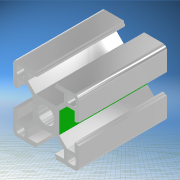
# Autodesk Inventor part: 30x30 aluminum
Saved by Autodesk Inventor 2020.2 (Build 242310000, 310)
## iProperties
Created: 2019-10-26
Part Number: 30x30 aluminum
Material: Aluminum 6061
Document SubType Name: Modeling
Designer: Sunoj
Density: 2.7 g/cm^3
Appearance: Aluminum - Flat
Mass: 340.698 g
Surface Area: 1270.55 cm^2
Volume: 126.184 cm^3
d0: 40.000 mm
Author: Sunoj
Autodesk Inventor part; units mm, degrees
ref_plane "YZ Plane" through (0, 0, 0) normal (1, 0, 0) x (0, 1, 0)
ref_plane "XZ Plane" through (0, 0, 0) normal (0, 1, 0) x (-1, 0, 0)
ref_plane "XY Plane" through (0, 0, 0) normal (0, 0, 1) x (1, 0, 0)
sketch "Sketch1" plane through (0, 0, 0) normal (0, 0, 1) x (1, 0, 0)
  line L0 (-4.1, 13) -> (-4.1, 14)
  line L1 (-4.1, 14) -> (-4.6, 14)
  line L2 (-4.6, 14) -> (-4.6, 15)
  line L3 (-4.6, 14) -> (-4.6, 15)
  line L4 (-4.6, 15) -> (-13, 15)
  arc A0 (-13, 15) -> (-15, 13) centre (-13, 13) ccw
  line L5 (-15, 13) -> (-15, 4.6)
  line L6 (-15, 13) -> (-15, 4.6)
  line L7 (-15, 4.6) -> (-14, 4.6)
  line L8 (-15, 4.6) -> (-14, 4.6)
  line L9 (-14, 4.6) -> (-14, 4.1)
  line L10 (-14, 4.6) -> (-14, 4.1)
  line L11 (-14, 4.1) -> (-13, 4.1)
  line L12 (-13, 4.1) -> (-13, 8.25)
  line L13 (-13, 8.25) -> (-9.5, 8.25)
  line L14 (-13, 8.25) -> (-9.5, 8.25)
  line L15 (-9.5, 8.25) -> (-6, 4.75)
  line L16 (-6, 4.75) -> (-6, -4.75)
  line L17 (-6, 4.75) -> (-6, -4.75)
  line L18 (-6, -4.75) -> (-9.5, -8.25)
  line L19 (-14, -4.1) -> (-13, -4.1)
  line L20 (-13, -4.1) -> (-14, -4.1)
  line L21 (-14, -4.6) -> (-14, -4.1)
  line L22 (-14, -4.1) -> (-14, -4.6)
  line L23 (-15, -4.6) -> (-14, -4.6)
  line L24 (-14, -4.6) -> (-15, -4.6)
  line L25 (-8.25, 13) -> (-4.1, 13)
  line L26 (-4.1, 13) -> (-8.25, 13)
  line L27 (-8.25, 9.5) -> (-8.25, 13)
  line L28 (-8.25, 13) -> (-8.25, 9.5)
  line L29 (-4.75, 6) -> (-8.25, 9.5)
  line L30 (-8.25, 9.5) -> (-4.75, 6)
  line L31 (4.75, 6) -> (-4.75, 6)
  line L32 (-4.75, 6) -> (4.75, 6)
  line L33 (4.75, 6) -> (8.25, 9.5)
  line L34 (8.25, 13) -> (8.25, 9.5)
  line L35 (8.25, 9.5) -> (8.25, 13)
  line L36 (8.25, 13) -> (4.1, 13)
  line L37 (4.1, 13) -> (4.1, 14)
  line L38 (4.6, 14) -> (4.1, 14)
  line L39 (4.1, 14) -> (4.6, 14)
  line L40 (4.6, 15) -> (4.6, 14)
  line L41 (4.6, 14) -> (4.6, 15)
  line L42 (4.6, 15) -> (13.08, 15)
  line L43 (15, 4.6) -> (15, 13)
  line L44 (15, 13) -> (15, 4.6)
  line L45 (14, 4.6) -> (15, 4.6)
  line L46 (15, 4.6) -> (14, 4.6)
  line L47 (14, 4.6) -> (14, 4.1)
  line L48 (13, 4.1) -> (14, 4.1)
  line L49 (14, 4.1) -> (13, 4.1)
  line L50 (13, 4.1) -> (13, 8.25)
  line L51 (9.5, 8.25) -> (13, 8.25)
  line L52 (13, 8.25) -> (9.5, 8.25)
  line L53 (6, 4.75) -> (9.5, 8.25)
  line L54 (9.5, 8.25) -> (6, 4.75)
  line L55 (6, 4.75) -> (6, -4.75)
  circle A1 centre (0, 0) radius 3.75
  line L56 (0, 0) -> (7.2487, 0)
  arc A2 (15, 13) -> (13, 15) centre (13, 13) ccw
  arc A3 (15, 13) -> (13.08, 15) centre (12.9977, 12.9994) ccw
  line L57 (-9.5, -8.25) -> (-6, -4.75)
  line L58 (-8.25, -9.5) -> (-4.75, -6)
  line L59 (-4.75, -6) -> (-8.25, -9.5)
  line L60 (-4.1, -13) -> (-4.1, -14)
  line L61 (-4.1, -14) -> (-4.6, -14)
  line L62 (-8.25, -13) -> (-4.1, -13)
  line L63 (-4.1, -13) -> (-8.25, -13)
  line L64 (-8.25, -9.5) -> (-8.25, -13)
  line L65 (-8.25, -13) -> (-8.25, -9.5)
  line L66 (-13, -8.25) -> (-9.5, -8.25)
  line L67 (-13, -4.1) -> (-13, -8.25)
  line L68 (-4.6, -14) -> (-4.6, -15)
  line L69 (-4.6, -14) -> (-4.6, -15)
  line L70 (-4.6, -15) -> (-13, -15)
  line L71 (-14, -4.6) -> (-14, -4.1)
  line L72 (-14, -4.6) -> (-14, -4.1)
  line L73 (-14, -4.1) -> (-13, -4.1)
  line L74 (-15, -4.6) -> (-14, -4.6)
  line L75 (-15, -4.6) -> (-14, -4.6)
  line L76 (-15, -13) -> (-15, -4.6)
  line L77 (-15, -13) -> (-15, -4.6)
  arc A4 (-15, -13) -> (-13, -15) centre (-13, -13) ccw
  line L78 (-13, -8.25) -> (-9.5, -8.25)
  line L79 (8.25, -13) -> (8.25, -9.5)
  line L80 (8.25, -9.5) -> (8.25, -13)
  line L81 (9.5, -8.25) -> (13, -8.25)
  line L82 (13, -8.25) -> (9.5, -8.25)
  line L83 (15, -13) -> (15, -4.6)
  line L84 (15, -4.6) -> (15, -13)
  line L85 (13, -4.1) -> (13, -8.25)
  line L86 (13, -4.1) -> (14, -4.1)
  line L87 (14, -4.1) -> (13, -4.1)
  line L88 (14, -4.6) -> (14, -4.1)
  line L89 (14, -4.6) -> (15, -4.6)
  line L90 (15, -4.6) -> (14, -4.6)
  line L91 (4.75, -6) -> (8.25, -9.5)
  line L92 (6, -4.75) -> (9.5, -8.25)
  line L93 (9.5, -8.25) -> (6, -4.75)
  arc A5 (13, -15) -> (15, -13) centre (13, -13) ccw
  arc A6 (13.08, -15) -> (15, -13) centre (12.9977, -12.9994) ccw
  line L94 (8.25, -13) -> (4.1, -13)
  line L95 (4.1, -13) -> (4.1, -14)
  line L96 (4.6, -14) -> (4.1, -14)
  line L97 (4.1, -14) -> (4.6, -14)
  line L98 (4.6, -15) -> (4.6, -14)
  line L99 (4.6, -14) -> (4.6, -15)
  line L100 (4.6, -15) -> (13.08, -15)
  line L101 (4.75, -6) -> (-4.75, -6)
  line L102 (-4.75, -6) -> (4.75, -6)
  circle A7 centre (0, 0) radius 3.75
  line L103 (-12.5, 13.5) -> (-10.7, 13.5)
  line L104 (-12.5, 13.5) -> (-10.7, 13.5)
  line L105 (-9.7, 12.5) -> (-9.7, 10.7)
  line L106 (-9.7, 12.5) -> (-9.7, 10.7)
  line L107 (-10.7, 9.7) -> (-12.5, 9.7)
  line L108 (-10.7, 9.7) -> (-12.5, 9.7)
  line L109 (-13.5, 12.5) -> (-13.5, 10.7)
  line L110 (-13.5, 10.7) -> (-13.5, 12.5)
  line L111 (-13.5, 12.5) -> (-13.5, 10.7)
  arc A8 (-12.5, 13.5) -> (-13.5, 12.5) centre (-12.5, 12.5) ccw
  arc A9 (-13.5, 10.7) -> (-12.5, 9.7) centre (-12.5, 10.7) ccw
  arc A10 (-13.5, 10.7) -> (-12.5, 9.7) centre (-12.5, 10.7) ccw
  arc A11 (-10.7, 9.7) -> (-9.7, 10.7) centre (-10.7, 10.7) ccw
  arc A12 (-9.7, 12.5) -> (-10.7, 13.5) centre (-10.7, 12.5) ccw
  arc A13 (-9.7, 12.5) -> (-10.7, 13.5) centre (-10.7, 12.5) ccw
  line L112 (0, 0) -> (0, 6.5)
  arc A14 (9.7, 10.7) -> (10.7, 9.7) centre (10.7, 10.7) ccw
  line L113 (9.7, 12.5) -> (9.7, 10.7)
  arc A15 (10.7, 13.5) -> (9.7, 12.5) centre (10.7, 12.5) ccw
  arc A16 (10.7, 13.5) -> (9.7, 12.5) centre (10.7, 12.5) ccw
  line L114 (9.7, 12.5) -> (9.7, 10.7)
  line L115 (12.5, 13.5) -> (10.7, 13.5)
  line L116 (12.5, 13.5) -> (10.7, 13.5)
  line L117 (10.7, 9.7) -> (12.5, 9.7)
  line L118 (10.7, 9.7) -> (12.5, 9.7)
  arc A17 (12.5, 9.7) -> (13.5, 10.7) centre (12.5, 10.7) ccw
  arc A18 (12.5, 9.7) -> (13.5, 10.7) centre (12.5, 10.7) ccw
  line L119 (13.5, 12.5) -> (13.5, 10.7)
  line L120 (13.5, 10.7) -> (13.5, 12.5)
  line L121 (13.5, 12.5) -> (13.5, 10.7)
  arc A19 (13.5, 12.5) -> (12.5, 13.5) centre (12.5, 12.5) ccw
  arc A20 (-13.5, -12.5) -> (-12.5, -13.5) centre (-12.5, -12.5) ccw
  line L122 (-9.7, -12.5) -> (-9.7, -10.7)
  line L123 (-9.7, -12.5) -> (-9.7, -10.7)
  line L124 (-10.7, -9.7) -> (-12.5, -9.7)
  line L125 (-10.7, -9.7) -> (-12.5, -9.7)
  line L126 (-13.5, -12.5) -> (-13.5, -10.7)
  line L127 (-13.5, -10.7) -> (-13.5, -12.5)
  line L128 (-13.5, -12.5) -> (-13.5, -10.7)
  arc A21 (-12.5, -9.7) -> (-13.5, -10.7) centre (-12.5, -10.7) ccw
  arc A22 (-12.5, -9.7) -> (-13.5, -10.7) centre (-12.5, -10.7) ccw
  arc A23 (-9.7, -10.7) -> (-10.7, -9.7) centre (-10.7, -10.7) ccw
  line L129 (-12.5, -13.5) -> (-10.7, -13.5)
  line L130 (-12.5, -13.5) -> (-10.7, -13.5)
  arc A24 (-10.7, -13.5) -> (-9.7, -12.5) centre (-10.7, -12.5) ccw
  arc A25 (-10.7, -13.5) -> (-9.7, -12.5) centre (-10.7, -12.5) ccw
  line L131 (12.5, -13.5) -> (10.7, -13.5)
  line L132 (12.5, -13.5) -> (10.7, -13.5)
  line L133 (9.7, -12.5) -> (9.7, -10.7)
  line L134 (9.7, -12.5) -> (9.7, -10.7)
  arc A26 (9.7, -12.5) -> (10.7, -13.5) centre (10.7, -12.5) ccw
  arc A27 (9.7, -12.5) -> (10.7, -13.5) centre (10.7, -12.5) ccw
  line L135 (13.5, -10.7) -> (13.5, -12.5)
  line L136 (13.5, -12.5) -> (13.5, -10.7)
  line L137 (13.5, -12.5) -> (13.5, -10.7)
  arc A28 (12.5, -13.5) -> (13.5, -12.5) centre (12.5, -12.5) ccw
  arc A29 (13.5, -10.7) -> (12.5, -9.7) centre (12.5, -10.7) ccw
  arc A30 (13.5, -10.7) -> (12.5, -9.7) centre (12.5, -10.7) ccw
  arc A31 (10.7, -9.7) -> (9.7, -10.7) centre (10.7, -10.7) ccw
  line L138 (10.7, -9.7) -> (12.5, -9.7)
  line L139 (10.7, -9.7) -> (12.5, -9.7)
  point P0 (14.7321, -14)
  point P1 (14.7321, 14)
  point P2 (14.7321, 14)
  point P3 (14.7321, -14)
  constraints: 280 end point, 79 symmetric about line, 66 point on circle, 32 centre point, 18 perpendicular, 13 collinear, 4 point on line, 3 horizontal, 3 vertical, 2 tangent, 1 coincident, 1 parallel, 21 other
extrude "Extrusion1" add sketch "Sketch1" along normal blind 40 contours L25 L27 L29 L31 L112 A1 L56 L55 L92 L81 L85 L86 L88 L89 L83 A5 L100 L98 L96 L95 L94 L79 L91 L101 L58 L64 L62 L60 L61 L68 L70 A4 L76 L23 L21 L19 L67 L66 L18 L16 L15 L13 L12 L11 L9 L7 L5 A0 L4 L2 L1 L0 | L31 L33 L34 L36 L37 L38 L40 L42 A2 L43 L45 L47 L48 L50 L51 L53 L55 L56 A1 L112
body "Solid1"
